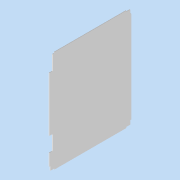
# Autodesk Inventor part: Acrly_Wand_1
Saved by Autodesk Inventor 2022 (Build 260153000, 153)
## iProperties
Created: 2021-12-15
Part Number: Acrly_Wand_1
Material: Generic
Document SubType Name: Modeling
Designer: Fabijansven
Density: 1 g/cm^3
Appearance: Default
Author: Fabijansven
Autodesk Inventor part; units mm, degrees
ref_plane "YZ Plane" through (0, 0, 0) normal (1, 0, 0) x (0, 1, 0)
ref_plane "XZ Plane" through (0, 0, 0) normal (0, 1, 0) x (-1, 0, 0)
ref_plane "XY Plane" through (0, 0, 0) normal (0, 0, 1) x (1, 0, 0)
sketch "Sketch1" plane through (0, 0, 0) normal (1, 0, 0) x (0, 1, 0)
  line L0 (0, 0) -> (822, 0)
  line L1 (822, 0) -> (822, -662)
  line L2 (822, -662) -> (0, -662)
  line L3 (0, -662) -> (0, 0)
  line L4 (822, 0) -> (814, 0)
  line L5 (814, 0) -> (814, -40)
  line L6 (814, -40) -> (822, -40)
  line L7 (822, -40) -> (822, 0)
  line L8 (822, 0) -> (782, 0)
  line L9 (782, 0) -> (782, -8)
  line L10 (782, -8) -> (822, -8)
  line L11 (822, -8) -> (822, 0)
  line L12 (856.5319, -331) -> (-65.1606, -331) construction
  line L13 (411, 165.682) -> (411, -1074.2454) construction
  line L14 (822, -662) -> (814, -662)
  line L15 (814, -662) -> (814, -622)
  line L16 (814, -622) -> (822, -622)
  line L17 (822, -622) -> (822, -662)
  line L18 (822, -662) -> (782, -662)
  line L19 (782, -662) -> (782, -654)
  line L20 (782, -654) -> (822, -654)
  line L21 (822, -654) -> (822, -662)
  line L22 (0, 0) -> (0, -662)
  line L23 (0, 0) -> (8, 0)
  line L24 (8, 0) -> (8, -40)
  line L25 (8, -40) -> (0, -40)
  line L26 (0, -40) -> (0, 0)
  line L27 (0, 0) -> (40, 0)
  line L28 (40, 0) -> (40, -8)
  line L29 (40, -8) -> (0, -8)
  line L30 (0, -8) -> (0, 0)
  line L31 (8, -622) -> (0, -622)
  line L32 (40, -654) -> (0, -654)
  line L33 (0, -662) -> (8, -662)
  line L34 (8, -662) -> (8, -622)
  line L35 (0, -622) -> (0, -662)
  line L36 (0, -662) -> (40, -662)
  line L37 (40, -662) -> (40, -654)
  line L38 (0, -654) -> (0, -662)
  point P0 (782, -662)
  point P1 (814, -654)
  point P2 (822, -40)
  point P3 (814, -8)
  point P4 (782, 0)
  point P5 (40, 0)
  point P6 (8, -8)
  point P7 (0, -40)
  point P8 (0, -622)
  point P9 (8, -654)
  dimension "d0" = 822
  dimension "d1" = 662
  dimension "d2" = 40
  dimension "d3" = 40
  dimension "d4" = 8
  dimension "d5" = 8
  dimension "d6" = 331
  dimension "d7" = 411
  constraints: 78 end point, 18 symmetric about line, 6 parallel, 4 horizontal, 3 perpendicular, 1 vertical
  measures "d0" distance of L1.end L2.end
  measures "d1" distance of L0.end L1.end
  measures "d2" distance of L4.end L5.end
  measures "d3" distance of L9.end L10.end
  measures "d4" distance of L8.end L9.end
  measures "d5" distance of L5.end L6.end
  measures "d6" distance between parallel lines of L0 L12
  measures "d7" distance between parallel lines of L3 L13
extrude "Extrusion1" add sketch "Sketch1" along normal blind 5 contours L0 L9 L10 L5 L6 L1 L16 L15 L20 L19 L2 L37 L32 L34 L31 L3 L25 L24 L29 L28
sketch "Sketch2" plane through (5, 0, 0) normal (1, 0, 0) x (0, 0, -1)
  line L0 (0, 136.35) -> (20.35, 136.35)
  line L1 (25.35, 141.35) -> (25.35, 251.35)
  line L2 (20.35, 256.35) -> (0, 256.35)
  line L3 (0, 256.35) -> (0, 136.35)
  line L4 (0, 782) -> (0, 40) projected
  line L5 (0, 696.35) -> (21.35, 696.35)
  line L6 (26.35, 701.35) -> (26.35, 816.35)
  line L7 (26.35, 816.35) -> (0, 816.35)
  line L8 (0, 816.35) -> (0, 696.35)
  line L9 (6.35, 816.35) -> (656.35, 816.35) projected
  line L10 (656.35, 6.35) -> (6.35, 6.35) projected
  arc A0 (21.35, 696.35) -> (26.35, 701.35) centre (21.35, 701.35) ccw
  arc A1 (20.35, 136.35) -> (25.35, 141.35) centre (20.35, 141.35) ccw
  arc A2 (25.35, 251.35) -> (20.35, 256.35) centre (20.35, 251.35) ccw
  point P0 (0, 0)
  point P1 (25.35, 256.35)
  point P2 (26.35, 696.35)
  dimension "d10" = 130
  dimension "d11" = 120
  dimension "d12" = 25.35
  dimension "d13" = 0
  dimension "d14" = 120
  dimension "d15" = 26.35
  dimension "d16" = 5
  constraints: 16 end point, 6 point on circle, 6 tangent, 5 point on line, 4 parallel, 3 centre point, 2 equal radius, 2 horizontal, 2 perpendicular, 1 collinear
  measures "d10" distance between parallel lines of L0 L10
  measures "d11" distance between parallel lines of L0 L2
  measures "d12" distance of point (25.35, 256.35) L2.end
  measures "d13" distance between parallel lines of L3 L4
  measures "d14" distance of point (26.35, 696.35) L6.end
  measures "d15" distance of L5.start point (26.35, 696.35)
  measures "d16" radius of A0
extrude "Extrusion2" cut sketch "Sketch2" against normal blind 10
equation "\"d6\" = 0.5 * d1"
equation "\"d7\" = 0.5 * d0"
body "Solid1"
